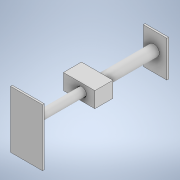
# Autodesk Inventor part: Деталь1
Saved by Autodesk Inventor 2020.1 (Build 241239000, 239)
## iProperties
Created: 2021-11-17
Part Number: Деталь1
Material: Типовые
Document SubType Name: Modeling
Designer: Ni3na
Density: 1 g/cm^3
Appearance: По умолчанию
Author: Ni3na
## iProperties of the stored document _3DПЕЧАТЬ.ipt
Created: 2021-12-12
Part Number: _3DПЕЧАТЬ
Material: Типовые
Document SubType Name: Modeling
Designer: User
Density: 1 g/cm^3
Appearance: По умолчанию
Author: User
Autodesk Inventor part; units mm, degrees
ref_plane "YZ Plane" through (0, 0, 0) normal (1, 0, 0) x (0, 1, 0)
ref_plane "XZ Plane" through (0, 0, 0) normal (0, 1, 0) x (-1, 0, 0)
ref_plane "XY Plane" through (0, 0, 0) normal (0, 0, 1) x (1, 0, 0)
sketch "Эскиз1" plane through (0, 0, 0) normal (0, 0, 1) x (1, 0, 0)
  circle A0 centre (-22.6267, 10.3807) radius 22.5037
  point P0 (0, 0)
  constraints: 1 centre point
extrude "Выдавливание1" add sketch "Эскиз1" along normal blind 500
sketch "Эскиз2" plane through (-22.6267, 10.3807, 0) normal (0, 0, -1) x (-1, 0, 0)
  circle A0 centre (0, 0) radius 25.8613
  circle A1 centre (0, 0) radius 29.6588
  point P0 (-22.6267, -10.3807)
  constraints: 2 centre point, 1 coincident
extrude "Выдавливание2" add sketch "Эскиз2" against normal mid plane 400
sketch "Эскиз3" plane through (-22.6267, 10.3807, -200) normal (0, 0, -1) x (-1, 0, 0)
  line L0 (58.9021, 92.5516) -> (-71.1943, 92.5516)
  line L1 (-71.1943, 92.5516) -> (-71.1943, -107.971)
  line L2 (-71.1943, -107.971) -> (58.9021, -107.971)
  line L3 (58.9021, -107.971) -> (58.9021, 92.5516)
  point P0 (-22.6267, -10.3807)
  constraints: 8 end point, 2 parallel, 1 horizontal, 1 perpendicular
extrude "Выдавливание3" add sketch "Эскиз3" along normal blind 10
sketch "Эскиз4" plane through (-22.6267, 10.3807, 500) normal (0, 0, 1) x (1, 0, 0)
  line L0 (-83.2061, -176.0697) -> (93.3264, -176.0697)
  line L1 (93.3264, -176.0697) -> (93.3264, 140.1274)
  line L2 (93.3264, 140.1274) -> (-83.2061, 140.1274)
  line L3 (-83.2061, 140.1274) -> (-83.2061, -176.0697)
  point P0 (22.6267, -10.3807)
  constraints: 8 end point, 2 parallel, 1 horizontal, 1 perpendicular
extrude "Выдавливание4" add sketch "Эскиз4" along normal blind 10
sketch "Эскиз5" plane through (-22.6267, 10.3807, 200) normal (0, 0, 1) x (1, 0, 0)
  line L0 (73.0581, -44.2251) -> (-101.1901, -44.2251)
  line L1 (-101.1901, -44.2251) -> (-101.1901, 42.3964)
  line L2 (-101.1901, 42.3964) -> (73.0581, 42.3964)
  line L3 (73.0581, 42.3964) -> (73.0581, -44.2251)
  circle A0 centre (0, 0) radius 25.8613 projected
  circle A1 centre (0, 0) radius 25.8613
  point P0 (22.6267, -10.3807)
  constraints: 8 end point, 2 parallel, 1 centre point, 1 coincident, 1 horizontal, 1 perpendicular
extrude "Выдавливание5" add sketch "Эскиз5" against normal blind 100
